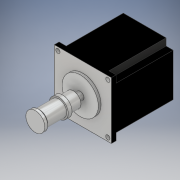
# Autodesk Inventor part: Motor
Saved by Autodesk Inventor 2019 (Build 230136000, 136)
## iProperties
Created: 2018-09-20
Part Number: Motor
Material: Generisch
Document SubType Name: Modeling
Designer: nico-
Density: 1 g/cm^3
Appearance: Vorgabe
Author: nico-
Autodesk Inventor part; units mm, degrees
ref_plane "XZ Plane" through (0, 0, 0) normal (0, 1, 0) x (-1, 0, 0)
ref_plane "XY Plane" through (0, 0, 0) normal (0, 0, 1) x (1, 0, 0)
sketch "Skizze1" plane through (0, 0, 0) normal (0, 0, 1) x (1, 0, 0)
  line L0 (0, 0) -> (60, 0)
  line L1 (60, 0) -> (60, 60)
  line L2 (60, 60) -> (0, 60)
  line L3 (0, 60) -> (0, 0)
  dimension "d0" = 60
  dimension "d1" = 60
  constraints: 8 end point, 2 parallel, 1 horizontal, 1 perpendicular
  measures "d0" distance of L2.end L1.end
  measures "d1" distance of L1.end L0.end
extrude "Extrusion1" add sketch "Skizze1" along normal blind 65
sketch "Skizze2" plane through (0, 0, 65) normal (0, 0, 1) x (1, 0, 0)
  circle A0 centre (30, 30) radius 4
  line L0 (0, 0) -> (60, 0) projected
  line L1 (0, 60) -> (0, 0) projected
  dimension "d4" = 8
  dimension "d10" = 30
  dimension "d11" = 30
  constraints: 1 centre point
  measures "d4" diameter of A0
  measures "d10" distance from line of L0 A0.centre
  measures "d11" distance from line of L1 A0.centre
extrude "Extrusion2" add sketch "Skizze2" along normal blind 10
ref_plane "Arbeitsebene1" through (30, 0, 0) normal (1, 0, 0) x (0, 1, 0)
sketch "Skizze5" plane through (30, 0, 0) normal (1, 0, 0) x (0, 1, 0)
  line L0 (34, 75) -> (26, 75) projected
  line L1 (30, 75) -> (30, 115)
  line L2 (30, 115) -> (40, 115)
  line L3 (40, 115) -> (40, 112)
  line L4 (38.375, 110.375) -> (40, 112)
  line L5 (38.375, 110.375) -> (38.375, 90.375)
  line L6 (38.375, 90.375) -> (40, 90.375)
  line L7 (40, 90.375) -> (40, 86.375)
  line L8 (40, 86.375) -> (38, 86.375)
  line L9 (38, 86.375) -> (38, 75)
  line L10 (38, 75) -> (30, 75)
  point P0 (0, 0)
  dimension "d25" = 40
  dimension "d26" = 10
  dimension "d27" = 3
  dimension "d30" = 1.625
  dimension "d31" = 135
  dimension "d32" = 20
  dimension "d33" = 4
  dimension "d34" = 2
  constraints: 20 end point, 5 perpendicular, 3 vertical, 1 horizontal, 1 midpoint
  measures "d25" distance of L1.start L1.end
  measures "d26" distance of L1.end L2.end
  measures "d27" distance of L2.end L3.end
  measures "d30" horizontal distance of L4.start L3.end
  measures "d31" angle of L4 L3
  measures "d32" distance of L4.start L5.end
  measures "d33" distance of L6.end L7.end
  measures "d34" distance of L7.end L8.end
revolve "Umdrehung1" add sketch "Skizze5" angle 360 about axis through (30, 30, 75) along (0, 0, 1)
sketch "Skizze6" plane through (0, 0, 0) normal (0, 0, -1) x (-1, 0, 0)
  line L0 (0, 0) -> (-60, 0) projected
  line L1 (0, 0) -> (-7.5, 0)
  line L2 (-7.5, 0) -> (-7.5, 7.5)
  line L3 (-7.5, 7.5) -> (0, 7.5)
  line L4 (0, 7.5) -> (0, 0)
  line L5 (-60, 0) -> (-52.5, 0)
  line L6 (-52.5, 0) -> (-52.5, 7.5)
  line L7 (-52.5, 7.5) -> (-60, 7.5)
  line L8 (-60, 7.5) -> (-60, 0)
  line L9 (-60, 60) -> (0, 60) projected
  line L10 (-60, 60) -> (-52.5, 60)
  line L11 (-52.5, 60) -> (-52.5, 52.5)
  line L12 (-52.5, 52.5) -> (-60, 52.5)
  line L13 (-60, 52.5) -> (-60, 60)
  line L14 (0, 60) -> (-7.5, 60)
  line L15 (-7.5, 60) -> (-7.5, 52.5)
  line L16 (-7.5, 52.5) -> (0, 52.5)
  line L17 (0, 52.5) -> (0, 60)
  dimension "d36" = 7.5
  dimension "d37" = 7.5
  dimension "d38" = 7.5
  dimension "d39" = 7.5
  dimension "d40" = 7.5
  dimension "d41" = 7.5
  dimension "d42" = 7.5
  dimension "d43" = 7.5
  constraints: 32 end point, 8 parallel, 4 horizontal, 4 perpendicular
  measures "d36" distance of L2.end L3.end
  measures "d37" distance of L1.end L2.end
  measures "d38" distance of L7.end L6.end
  measures "d39" distance of L6.end L5.end
  measures "d40" distance of L11.end L12.end
  measures "d41" distance of L10.end L11.end
  measures "d42" distance of L16.end L15.end
  measures "d43" distance of L15.end L14.end
extrude "Extrusion4" cut sketch "Skizze6" against normal blind 60
sketch "Skizze7" plane through (0, 0, 65) normal (0, 0, 1) x (1, 0, 0)
  circle A0 centre (3.75, 3.75) radius 2.25
  circle A1 centre (56.25, 3.75) radius 2.25
  circle A2 centre (56.25, 56.25) radius 2.25
  circle A3 centre (3.75, 56.25) radius 2.25
  point P0 (0, 0)
  dimension "d46" = 4.5
  dimension "d47" = 4.5
  dimension "d48" = 4.5
  dimension "d49" = 4.5
  constraints: 4 centre point
  measures "d46" diameter of A0
  measures "d47" diameter of A1
  measures "d48" diameter of A2
  measures "d49" diameter of A3
extrude "Extrusion5" cut sketch "Skizze7" against normal blind 5
sketch "Skizze8" plane through (0, 0, 65) normal (0, 0, 1) x (1, 0, 0)
  circle A0 centre (30, 30) radius 8 projected
  circle A1 centre (30, 30) radius 19.075
  point P0 (0, 0)
  dimension "d52" = 38.15
  constraints: 1 centre point, 1 coincident
  measures "d52" diameter of A1
extrude "Extrusion6" add sketch "Skizze8" along normal blind 2.8 contours A0 | A1
